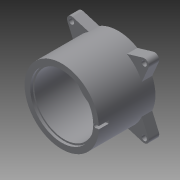
# Autodesk Inventor part: Nikon Mount 02
Saved by Autodesk Inventor 2013 (Build 170138000, 138)
## iProperties
Created: 2014-04-13
Part Number: Nikon Mount 02
Material: Generic
Document SubType Name: Modeling
Designer: spichelh
Density: 1 g/cm^3
Author: spichelh
Autodesk Inventor part; units mm, degrees
ref_plane "YZ Plane" through (0, 0, 0) normal (1, 0, 0) x (0, 1, 0)
ref_plane "XZ Plane" through (0, 0, 0) normal (0, 1, 0) x (-1, 0, 0)
ref_plane "XY Plane" through (0, 0, 0) normal (0, 0, 1) x (1, 0, 0)
sketch "Sketch1" plane through (0, 0, 0) normal (0, 0, 1) x (1, 0, 0)
  circle A0 centre (0.0056, 55.7001) radius 1.4
  arc A1 (1.0027, 59.055) -> (-3.2054, 54.3074) centre (0.0056, 55.7001) ccw
  circle A2 centre (27.9456, 30.9351) radius 20
  line L0 (27.9456, 30.9351) -> (77.9456, 30.9351) construction
  line L1 (27.9456, 30.9351) -> (77.9456, 30.9351) construction
  line L2 (1.0027, 59.055) -> (13.3178, 55.3948)
  line L3 (-3.2054, 54.3074) -> (1.9067, 42.5207)
  circle A3 centre (0.0056, 6.1701) radius 1.4
  circle A4 centre (55.8856, 6.1701) radius 1.4
  line L4 (55.8856, 55.7001) -> (0.0056, 6.1701) construction
  line L5 (55.8856, 6.1701) -> (0.0056, 55.7001) construction
  line L6 (27.9456, 30.9351) -> (27.9456, 40.8752) construction
  line L7 (27.9456, 30.9351) -> (19.6856, 30.9351) construction
  arc A5 (59.0966, 54.3074) -> (54.8884, 59.055) centre (55.8856, 55.7001) ccw
  line L8 (54.8884, 59.055) -> (42.5733, 55.3948)
  line L9 (59.0966, 54.3074) -> (53.9844, 42.5207)
  circle A6 centre (55.8856, 55.7001) radius 1.4
  arc A7 (42.5733, 55.3948) -> (13.3178, 55.3948) centre (27.9456, 30.9351) ccw
  arc A8 (1.9067, 42.5207) -> (53.9844, 42.5207) centre (27.9456, 30.9351) ccw construction
  arc A9 (42.5733, 55.3948) -> (13.3178, 55.3948) centre (27.9456, 30.9351) ccw construction
  arc A10 (-3.2054, 7.5627) -> (1.0027, 2.8151) centre (0.0056, 6.1701) ccw
  line L10 (1.0027, 2.8151) -> (13.3178, 6.4753)
  line L11 (-3.2054, 7.5627) -> (1.9067, 19.3494)
  arc A11 (54.8884, 2.8151) -> (59.0966, 7.5627) centre (55.8856, 6.1701) ccw
  line L12 (54.8884, 2.8151) -> (42.5733, 6.4753)
  line L13 (59.0966, 7.5627) -> (53.9844, 19.3494)
  arc A12 (53.9844, 19.3494) -> (53.9844, 42.5207) centre (27.9456, 30.9351) ccw
  arc A13 (1.9067, 42.5207) -> (1.9067, 19.3494) centre (27.9456, 30.9351) ccw
  arc A14 (13.3178, 6.4753) -> (42.5733, 6.4753) centre (27.9456, 30.9351) ccw
  point P0 (0, 0)
  point P1 (27.9456, 30.9351)
  dimension "d222" = 2.8
  dimension "d223" = 7
  dimension "d233" = 40
  dimension "d234" = 27.9456
  dimension "d291" = 55.88
  dimension "d292" = 49.53
  dimension "d293" = 2.8
  dimension "d294" = 2.8
  dimension "d295" = 155
  dimension "d296" = 155
  dimension "d298" = 30.9351
  dimension "d299" = 28.5
  dimension "d300" = 155
  dimension "d301" = 3.5
  dimension "d302" = 155
  dimension "d303" = 28.5
  constraints: 28 end point, 22 point on circle, 15 centre point, 10 symmetric about line, 6 coincident, 4 tangent, 2 horizontal, 2 horizontal alignment, 2 midpoint, 2 perpendicular, 2 vertical alignment, 3 other
  measures "d222" diameter of A0
  measures "d223" diameter of A1
  measures "d233" diameter of A2
  measures "d234" horizontal distance of L0.start point (0, 0)
  measures "d291" distance of A0.centre L4.start
  measures "d292" distance of point (0.006, 6.17) A0.centre
  measures "d293" diameter of A3
  measures "d294" diameter of A4
  measures "d295" angle of L5 L2
  measures "d296" angle of L5 L3
  measures "d298" vertical distance of point (0, 0) A8.centre
  measures "d299" radius of A7
  measures "d300" angle of L10 L4
  measures "d301" radius of A10
  measures "d302" angle of L4 L11
  measures "d303" radius of A12
extrude "Extrusion1" add sketch "Sketch1" along normal blind 8
sketch "Sketch14" plane through (0, 0, 8) normal (0, 0, 1) x (1, 0, 0)
  circle A0 centre (27.9456, 30.9351) radius 23
  line L0 (27.9493, 53.53) -> (27.94, -2.5) construction
  line L1 (50.88, 56.34) -> (5, 56.34) construction
  line L2 (-22.86, -0.81) -> (78.74, -0.81) construction
  line L3 (-22.86, 56.34) -> (-22.86, -0.81) construction
  line L4 (78.74, -0.81) -> (78.74, 56.34) construction
  circle A1 centre (27.9456, 30.9351) radius 20 projected
  arc A2 (42.5733, 55.3948) -> (13.3178, 55.3948) centre (27.9456, 30.9351) ccw projected
  circle A3 centre (27.9456, 30.9351) radius 28.5
  point P0 (52.88, -2.5)
  dimension "d96" = 46
  constraints: 2 centre point, 2 coincident, 2 end point, 1 concentric, 1 point on line
  measures "d96" diameter of A0
extrude "Extrusion14" add sketch "Sketch14" against normal blind 8 contours A3 A2
sketch "Sketch15" plane through (0, 0, 8) normal (0, 0, 1) x (1, 0, 0)
  circle A0 centre (27.9456, 30.9351) radius 20 projected
  circle A1 centre (27.9456, 30.9351) radius 28.5
  circle A2 centre (27.9456, 30.9351) radius 23
  dimension "d306" = 46
  dimension "d307" = 57
  constraints: 3 coincident, 2 centre point
  measures "d306" diameter of A2
  measures "d307" diameter of A1
extrude "Extrusion15" add sketch "Sketch15" along normal blind 35.44 contours A1
sketch "Sketch41" plane through (0, 0, 8) normal (0, 0, 1) x (1, 0, 0)
  arc A0 (55.6663, 24.3163) -> (0.2017, 24.4136) centre (27.94, 27.765) ccw projected
  circle A1 centre (0.0056, 55.7001) radius 1.4 projected
  circle A2 centre (0.0056, 55.7001) radius 2
  line L0 (27.94, 27.765) -> (27.94, 38.7432) construction
  line L1 (27.94, 27.765) -> (35.7476, 27.765) construction
  circle A3 centre (55.8744, 55.7001) radius 2
  circle A4 centre (0.0056, 6.1701) radius 1.4 projected
  circle A5 centre (55.8856, 6.1701) radius 1.4 projected
  circle A6 centre (0.0056, 6.1701) radius 2
  circle A7 centre (55.8856, 6.1701) radius 2
  point P0 (3.5123, 41.3272)
  point P1 (14.3575, 52.1814)
  point P2 (0, 0)
  dimension "d287" = 4
  dimension "d304" = 4
  dimension "d305" = 4
  constraints: 4 centre point, 4 end point, 3 coincident, 1 perpendicular, 1 symmetric about line, 1 vertical, 1 other
  measures "d287" diameter of A2
  measures "d304" diameter of A6
  measures "d305" diameter of A7
extrude "Extrusion39" cut sketch "Sketch41" against normal blind 4 contours A1 | A2 | A3 | A4 | A6 | A7
sketch "Sketch17" plane through (0, 0, 0) normal (0, 0, -1) x (-1, 0, 0)
  line L0 (-37.3456, 38.9851) -> (-18.5456, 38.9851)
  line L1 (-17.5456, 37.9851) -> (-17.5456, 23.8851)
  line L2 (-18.5456, 22.8851) -> (-37.3456, 22.8851)
  line L3 (-38.3456, 23.8851) -> (-38.3456, 37.9851)
  line L4 (-17.5456, 38.9851) -> (-38.3456, 22.8851) construction
  line L5 (-17.5456, 22.8851) -> (-38.3456, 38.9851) construction
  circle A0 centre (-27.9456, 30.9351) radius 23
  arc A1 (-37.3456, 38.9851) -> (-38.3456, 37.9851) centre (-37.3456, 37.9851) ccw
  arc A2 (-38.3456, 23.8851) -> (-37.3456, 22.8851) centre (-37.3456, 23.8851) ccw
  arc A3 (-18.5456, 22.8851) -> (-17.5456, 23.8851) centre (-18.5456, 23.8851) ccw
  arc A4 (-17.5456, 37.9851) -> (-18.5456, 38.9851) centre (-18.5456, 37.9851) ccw
  circle A5 centre (-27.9456, 30.9351) radius 20 projected
  point P0 (0, 0)
  point P1 (-27.9456, 30.9351)
  dimension "d111" = 20.8
  dimension "d112" = 16.1
  dimension "d115" = 1
  dimension "d308" = 46
  constraints: 12 end point, 8 point on circle, 8 point on line, 8 tangent, 5 centre point, 3 equal radius, 2 coincident, 2 midpoint, 2 parallel, 1 horizontal, 1 perpendicular
  measures "d111" distance of L5.start L4.end
  measures "d112" distance of L4.start L5.start
  measures "d115" radius of A1
  measures "d308" diameter of A0
extrude "Extrusion17" add sketch "Sketch17" against normal blind 11 contours A0 | A5
sketch "Sketch18" plane through (27.94, 27.765, 11) normal (0, 0, 1) x (1, 0, 0)
  line L0 (10.4056, 10.2201) -> (10.4056, -3.8799) projected
  line L1 (9.4056, -4.8799) -> (-9.3944, -4.8799) projected
  line L2 (-10.3944, -3.8799) -> (-10.3944, 10.2201) projected
  line L3 (-9.3944, 11.2201) -> (9.4056, 11.2201) projected
  arc A0 (10.4056, 10.2201) -> (9.4056, 11.2201) centre (9.4056, 10.2201) ccw projected
  arc A1 (9.4056, -4.8799) -> (10.4056, -3.8799) centre (9.4056, -3.8799) ccw projected
  arc A2 (-10.3944, -3.8799) -> (-9.3944, -4.8799) centre (-9.3944, -3.8799) ccw projected
  arc A3 (-9.3944, 11.2201) -> (-10.3944, 10.2201) centre (-9.3944, 10.2201) ccw projected
  line L4 (9.4056, 12.2201) -> (-9.3944, 12.2201)
  arc A4 (-9.3944, 12.2201) -> (-11.3944, 10.2201) centre (-9.3944, 10.2201) ccw
  line L5 (-11.3944, 10.2201) -> (-11.3944, -3.8799)
  arc A5 (-11.3944, -3.8799) -> (-9.3944, -5.8799) centre (-9.3944, -3.8799) ccw
  line L6 (-9.3944, -5.8799) -> (9.4056, -5.8799)
  arc A6 (9.4056, -5.8799) -> (11.4056, -3.8799) centre (9.4056, -3.8799) ccw
  line L7 (11.4056, -3.8799) -> (11.4056, 10.2201)
  arc A7 (11.4056, 10.2201) -> (9.4056, 12.2201) centre (9.4056, 10.2201) ccw
  point P0 (10.4, 8.05)
  point P1 (10.4, -8.05)
  point P2 (-10.4, -8.05)
  point P3 (-10.4, 8.05)
  point P4 (-27.94, -27.765)
  dimension "d116" = 1
  constraints: 8 end point, 8 point on circle, 4 centre point, 11 other
extrude "Extrusion18" cut sketch "Sketch18" against normal blind 8
sketch "Sketch19" plane through (27.94, 27.765, 11) normal (0, 0, 1) x (1, 0, 0)
  arc A0 (-9.3944, 12.2201) -> (-11.3944, 10.2201) centre (-9.3944, 10.2201) ccw projected
  line L0 (-9.3944, 12.2201) -> (9.4056, 12.2201) projected
  arc A1 (11.4056, 10.2201) -> (9.4056, 12.2201) centre (9.4056, 10.2201) ccw projected
  line L1 (11.4056, 10.2201) -> (11.4056, -3.8799) projected
  arc A2 (9.4056, -5.8799) -> (11.4056, -3.8799) centre (9.4056, -3.8799) ccw projected
  line L2 (9.4056, -5.8799) -> (-9.3944, -5.8799) projected
  arc A3 (-11.3944, -3.8799) -> (-9.3944, -5.8799) centre (-9.3944, -3.8799) ccw projected
  line L3 (-11.3944, -3.8799) -> (-11.3944, 10.2201) projected
  line L4 (9.4056, 13.2201) -> (-9.3944, 13.2201)
  arc A4 (-9.3944, 13.2201) -> (-12.3944, 10.2201) centre (-9.3944, 10.2201) ccw
  line L5 (-12.3944, 10.2201) -> (-12.3944, -3.8799)
  arc A5 (-12.3944, -3.8799) -> (-9.3944, -6.8799) centre (-9.3944, -3.8799) ccw
  line L6 (-9.3944, -6.8799) -> (9.4056, -6.8799)
  arc A6 (9.4056, -6.8799) -> (12.4056, -3.8799) centre (9.4056, -3.8799) ccw
  line L7 (12.4056, -3.8799) -> (12.4056, 10.2201)
  arc A7 (12.4056, 10.2201) -> (9.4056, 13.2201) centre (9.4056, 10.2201) ccw
  point P0 (-27.94, -27.765)
  dimension "d119" = 1
  constraints: 8 end point, 8 point on circle, 4 centre point, 7 other
  measures "d119" distance between parallel lines of L0 L4
extrude "Extrusion19" cut sketch "Sketch19" against normal blind 7
sketch "Sketch20" plane through (27.94, 27.765, 11) normal (0, 0, 1) x (1, 0, 0)
  arc A0 (-9.3944, 13.2201) -> (-12.3944, 10.2201) centre (-9.3944, 10.2201) ccw projected
  line L0 (-9.3944, 13.2201) -> (9.4056, 13.2201) projected
  arc A1 (12.4056, 10.2201) -> (9.4056, 13.2201) centre (9.4056, 10.2201) ccw projected
  line L1 (12.4056, 10.2201) -> (12.4056, -3.8799) projected
  arc A2 (9.4056, -6.8799) -> (12.4056, -3.8799) centre (9.4056, -3.8799) ccw projected
  line L2 (9.4056, -6.8799) -> (-9.3944, -6.8799) projected
  arc A3 (-12.3944, -3.8799) -> (-9.3944, -6.8799) centre (-9.3944, -3.8799) ccw projected
  line L3 (-12.3944, -3.8799) -> (-12.3944, 10.2201) projected
  line L4 (9.4056, 14.2201) -> (-9.3944, 14.2201)
  arc A4 (-9.3944, 14.2201) -> (-13.3944, 10.2201) centre (-9.3944, 10.2201) ccw
  line L5 (-13.3944, 10.2201) -> (-13.3944, -3.8799)
  arc A5 (-13.3944, -3.8799) -> (-9.3944, -7.8799) centre (-9.3944, -3.8799) ccw
  line L6 (-9.3944, -7.8799) -> (9.4056, -7.8799)
  arc A6 (9.4056, -7.8799) -> (13.4056, -3.8799) centre (9.4056, -3.8799) ccw
  line L7 (13.4056, -3.8799) -> (13.4056, 10.2201)
  arc A7 (13.4056, 10.2201) -> (9.4056, 14.2201) centre (9.4056, 10.2201) ccw
  point P0 (-27.94, -27.765)
  dimension "d122" = 1
  constraints: 8 end point, 8 point on circle, 4 centre point, 7 other
  measures "d122" distance between parallel lines of L4 L0
extrude "Extrusion20" cut sketch "Sketch20" against normal blind 6
sketch "Sketch21" plane through (27.94, 27.765, 11) normal (0, 0, 1) x (1, 0, 0)
  arc A0 (-9.3944, 14.2201) -> (-13.3944, 10.2201) centre (-9.3944, 10.2201) ccw projected
  line L0 (-9.3944, 14.2201) -> (9.4056, 14.2201) projected
  arc A1 (13.4056, 10.2201) -> (9.4056, 14.2201) centre (9.4056, 10.2201) ccw projected
  line L1 (13.4056, 10.2201) -> (13.4056, -3.8799) projected
  arc A2 (9.4056, -7.8799) -> (13.4056, -3.8799) centre (9.4056, -3.8799) ccw projected
  line L2 (9.4056, -7.8799) -> (-9.3944, -7.8799) projected
  arc A3 (-13.3944, -3.8799) -> (-9.3944, -7.8799) centre (-9.3944, -3.8799) ccw projected
  line L3 (-13.3944, -3.8799) -> (-13.3944, 10.2201) projected
  line L4 (9.4056, 15.2201) -> (-9.3944, 15.2201)
  arc A4 (-9.3944, 15.2201) -> (-14.3944, 10.2201) centre (-9.3944, 10.2201) ccw
  line L5 (-14.3944, 10.2201) -> (-14.3944, -3.8799)
  arc A5 (-14.3944, -3.8799) -> (-9.3944, -8.8799) centre (-9.3944, -3.8799) ccw
  line L6 (-9.3944, -8.8799) -> (9.4056, -8.8799)
  arc A6 (9.4056, -8.8799) -> (14.4056, -3.8799) centre (9.4056, -3.8799) ccw
  line L7 (14.4056, -3.8799) -> (14.4056, 10.2201)
  arc A7 (14.4056, 10.2201) -> (9.4056, 15.2201) centre (9.4056, 10.2201) ccw
  point P0 (-27.94, -27.765)
  dimension "d125" = 1
  constraints: 8 end point, 8 point on circle, 4 centre point, 7 other
  measures "d125" distance between parallel lines of L0 L4
extrude "Extrusion21" cut sketch "Sketch21" against normal blind 5
sketch "Sketch22" plane through (27.94, 27.765, 11) normal (0, 0, 1) x (1, 0, 0)
  arc A0 (-9.3944, 15.2201) -> (-14.3944, 10.2201) centre (-9.3944, 10.2201) ccw projected
  line L0 (-9.3944, 15.2201) -> (9.4056, 15.2201) projected
  arc A1 (14.4056, 10.2201) -> (9.4056, 15.2201) centre (9.4056, 10.2201) ccw projected
  line L1 (14.4056, 10.2201) -> (14.4056, -3.8799) projected
  arc A2 (9.4056, -8.8799) -> (14.4056, -3.8799) centre (9.4056, -3.8799) ccw projected
  line L2 (9.4056, -8.8799) -> (-9.3944, -8.8799) projected
  arc A3 (-14.3944, -3.8799) -> (-9.3944, -8.8799) centre (-9.3944, -3.8799) ccw projected
  line L3 (-14.3944, -3.8799) -> (-14.3944, 10.2201) projected
  line L4 (9.4056, 16.2201) -> (-9.3944, 16.2201)
  arc A4 (-9.3944, 16.2201) -> (-15.3944, 10.2201) centre (-9.3944, 10.2201) ccw
  line L5 (-15.3944, 10.2201) -> (-15.3944, -3.8799)
  arc A5 (-15.3944, -3.8799) -> (-9.3944, -9.8799) centre (-9.3944, -3.8799) ccw
  line L6 (-9.3944, -9.8799) -> (9.4056, -9.8799)
  arc A6 (9.4056, -9.8799) -> (15.4056, -3.8799) centre (9.4056, -3.8799) ccw
  line L7 (15.4056, -3.8799) -> (15.4056, 10.2201)
  arc A7 (15.4056, 10.2201) -> (9.4056, 16.2201) centre (9.4056, 10.2201) ccw
  point P0 (-27.94, -27.765)
  dimension "d128" = 1
  constraints: 8 end point, 8 point on circle, 4 centre point, 7 other
  measures "d128" distance between parallel lines of L0 L4
extrude "Extrusion22" cut sketch "Sketch22" against normal blind 4
sketch "Sketch23" plane through (27.94, 27.765, 11) normal (0, 0, 1) x (1, 0, 0)
  arc A0 (-9.3944, 16.2201) -> (-15.3944, 10.2201) centre (-9.3944, 10.2201) ccw projected
  line L0 (-9.3944, 16.2201) -> (9.4056, 16.2201) projected
  arc A1 (15.4056, 10.2201) -> (9.4056, 16.2201) centre (9.4056, 10.2201) ccw projected
  line L1 (15.4056, 10.2201) -> (15.4056, -3.8799) projected
  arc A2 (9.4056, -9.8799) -> (15.4056, -3.8799) centre (9.4056, -3.8799) ccw projected
  line L2 (9.4056, -9.8799) -> (-9.3944, -9.8799) projected
  arc A3 (-15.3944, -3.8799) -> (-9.3944, -9.8799) centre (-9.3944, -3.8799) ccw projected
  line L3 (-15.3944, -3.8799) -> (-15.3944, 10.2201) projected
  line L4 (9.4056, 17.2201) -> (-9.3944, 17.2201)
  arc A4 (-9.3944, 17.2201) -> (-16.3944, 10.2201) centre (-9.3944, 10.2201) ccw
  line L5 (-16.3944, 10.2201) -> (-16.3944, -3.8799)
  arc A5 (-16.3944, -3.8799) -> (-9.3944, -10.8799) centre (-9.3944, -3.8799) ccw
  line L6 (-9.3944, -10.8799) -> (9.4056, -10.8799)
  arc A6 (9.4056, -10.8799) -> (16.4056, -3.8799) centre (9.4056, -3.8799) ccw
  line L7 (16.4056, -3.8799) -> (16.4056, 10.2201)
  arc A7 (16.4056, 10.2201) -> (9.4056, 17.2201) centre (9.4056, 10.2201) ccw
  point P0 (-27.94, -27.765)
  dimension "d131" = 1
  constraints: 8 end point, 8 point on circle, 4 centre point, 7 other
  measures "d131" distance between parallel lines of L0 L4
extrude "Extrusion23" cut sketch "Sketch23" against normal blind 3
sketch "Sketch24" plane through (27.94, 27.765, 11) normal (0, 0, 1) x (1, 0, 0)
  arc A0 (-9.3944, 17.2201) -> (-16.3944, 10.2201) centre (-9.3944, 10.2201) ccw projected
  line L0 (-9.3944, 17.2201) -> (9.4056, 17.2201) projected
  arc A1 (16.4056, 10.2201) -> (9.4056, 17.2201) centre (9.4056, 10.2201) ccw projected
  line L1 (16.4056, 10.2201) -> (16.4056, -3.8799) projected
  arc A2 (9.4056, -10.8799) -> (16.4056, -3.8799) centre (9.4056, -3.8799) ccw projected
  line L2 (9.4056, -10.8799) -> (-9.3944, -10.8799) projected
  arc A3 (-16.3944, -3.8799) -> (-9.3944, -10.8799) centre (-9.3944, -3.8799) ccw projected
  line L3 (-16.3944, -3.8799) -> (-16.3944, 10.2201) projected
  line L4 (9.4056, 18.2201) -> (-9.3944, 18.2201)
  arc A4 (-9.3944, 18.2201) -> (-17.3944, 10.2201) centre (-9.3944, 10.2201) ccw
  line L5 (-17.3944, 10.2201) -> (-17.3944, -3.8799)
  arc A5 (-17.3944, -3.8799) -> (-9.3944, -11.8799) centre (-9.3944, -3.8799) ccw
  line L6 (-9.3944, -11.8799) -> (9.4056, -11.8799)
  arc A6 (9.4056, -11.8799) -> (17.4056, -3.8799) centre (9.4056, -3.8799) ccw
  line L7 (17.4056, -3.8799) -> (17.4056, 10.2201)
  arc A7 (17.4056, 10.2201) -> (9.4056, 18.2201) centre (9.4056, 10.2201) ccw
  point P0 (-27.94, -27.765)
  dimension "d134" = 1
  constraints: 8 end point, 8 point on circle, 4 centre point, 7 other
  measures "d134" distance between parallel lines of L0 L4
extrude "Extrusion24" cut sketch "Sketch24" against normal blind 2
sketch "Sketch25" plane through (27.94, 27.765, 11) normal (0, 0, 1) x (1, 0, 0)
  arc A0 (-9.3944, 18.2201) -> (-17.3944, 10.2201) centre (-9.3944, 10.2201) ccw projected
  line L0 (-9.3944, 18.2201) -> (9.4056, 18.2201) projected
  arc A1 (17.4056, 10.2201) -> (9.4056, 18.2201) centre (9.4056, 10.2201) ccw projected
  line L1 (17.4056, 10.2201) -> (17.4056, -3.8799) projected
  arc A2 (9.4056, -11.8799) -> (17.4056, -3.8799) centre (9.4056, -3.8799) ccw projected
  line L2 (9.4056, -11.8799) -> (-9.3944, -11.8799) projected
  arc A3 (-17.3944, -3.8799) -> (-9.3944, -11.8799) centre (-9.3944, -3.8799) ccw projected
  line L3 (-17.3944, -3.8799) -> (-17.3944, 10.2201) projected
  line L4 (9.4056, 19.2201) -> (-9.3944, 19.2201)
  arc A4 (-9.3944, 19.2201) -> (-18.3944, 10.2201) centre (-9.3944, 10.2201) ccw
  line L5 (-18.3944, 10.2201) -> (-18.3944, -3.8799)
  arc A5 (-18.3944, -3.8799) -> (-9.3944, -12.8799) centre (-9.3944, -3.8799) ccw
  line L6 (-9.3944, -12.8799) -> (9.4056, -12.8799)
  arc A6 (9.4056, -12.8799) -> (18.4056, -3.8799) centre (9.4056, -3.8799) ccw
  line L7 (18.4056, -3.8799) -> (18.4056, 10.2201)
  arc A7 (18.4056, 10.2201) -> (9.4056, 19.2201) centre (9.4056, 10.2201) ccw
  point P0 (-27.94, -27.765)
  dimension "d137" = 1
  constraints: 8 end point, 8 point on circle, 4 centre point, 7 other
  measures "d137" distance between parallel lines of L0 L4
extrude "Extrusion25" cut sketch "Sketch25" against normal blind 1
sketch "Sketch39" plane through (0, 0, 0) normal (0, 0, -1) x (-1, 0, 0)
  arc A0 (-38.3456, 23.8851) -> (-37.3456, 22.8851) centre (-37.3456, 23.8851) ccw projected
  line L0 (-38.3456, 23.8851) -> (-38.3456, 37.9851) projected
  arc A1 (-37.3456, 38.9851) -> (-38.3456, 37.9851) centre (-37.3456, 37.9851) ccw projected
  line L1 (-37.3456, 38.9851) -> (-18.5456, 38.9851) projected
  arc A2 (-17.5456, 37.9851) -> (-18.5456, 38.9851) centre (-18.5456, 37.9851) ccw projected
  line L2 (-17.5456, 37.9851) -> (-17.5456, 23.8851) projected
  arc A3 (-18.5456, 22.8851) -> (-17.5456, 23.8851) centre (-18.5456, 23.8851) ccw projected
  line L3 (-18.5456, 22.8851) -> (-37.3456, 22.8851) projected
  line L4 (-40.4456, 43.4351) -> (-15.4456, 43.4351)
  line L5 (-15.4456, 43.4351) -> (-15.4456, 18.4351)
  line L6 (-15.4456, 18.4351) -> (-40.4456, 18.4351)
  line L7 (-40.4456, 18.4351) -> (-40.4456, 43.4351)
  line L8 (-15.4456, 43.4351) -> (-40.4456, 18.4351) construction
  line L9 (-40.4456, 43.4351) -> (-15.4456, 18.4351) construction
  line L10 (-18.5456, 23.8851) -> (-37.3456, 37.9851) construction
  line L11 (-37.3456, 23.8851) -> (-18.5456, 37.9851) construction
  point P0 (-27.9456, 30.9351)
  dimension "d217" = 25
  dimension "d219" = 25
  constraints: 16 end point, 3 midpoint, 2 parallel, 1 horizontal, 1 perpendicular
  measures "d217" distance of L4.start L4.end
  measures "d219" distance of L4.end L5.end
extrude "Extrusion38" cut sketch "Sketch39" against normal blind 1.6
sketch "Sketch40" plane through (0, 0, 1.6) normal (0, 0, -1) x (-1, 0, 0)
  line L0 (-37.3456, 22.8851) -> (-18.5456, 22.8851) projected
  arc A0 (-38.3456, 23.8851) -> (-37.3456, 22.8851) centre (-37.3456, 23.8851) ccw projected
  line L1 (-38.3456, 37.9851) -> (-38.3456, 23.8851) projected
  arc A1 (-37.3456, 38.9851) -> (-38.3456, 37.9851) centre (-37.3456, 37.9851) ccw projected
  line L2 (-18.5456, 38.9851) -> (-37.3456, 38.9851) projected
  arc A2 (-17.5456, 37.9851) -> (-18.5456, 38.9851) centre (-18.5456, 37.9851) ccw projected
  line L3 (-17.5456, 23.8851) -> (-17.5456, 37.9851) projected
  arc A3 (-18.5456, 22.8851) -> (-17.5456, 23.8851) centre (-18.5456, 23.8851) ccw projected
  line L4 (-40.4456, 43.4351) -> (-15.4456, 43.4351) projected
  line L5 (-40.4456, 18.4351) -> (-40.4456, 43.4351) projected
  line L6 (-15.4456, 18.4351) -> (-40.4456, 18.4351) projected
  line L7 (-15.4456, 43.4351) -> (-15.4456, 18.4351) projected
  line L8 (-15.4456, 43.4351) -> (-40.4456, 18.4351) construction
  line L9 (-15.4456, 18.4351) -> (-40.4456, 43.4351) construction
  point P0 (0, 0)
  point P1 (-27.9456, 30.9351)
  constraints: 4 end point, 1 midpoint, 1 perpendicular
sketch "Sketch42" plane through (27.9456, 30.9351, 43.44) normal (0, 0, 1) x (1, 0, 0)
  circle A0 centre (0, 0) radius 23 projected
  circle A1 centre (0, 0) radius 28.5 projected
  circle A2 centre (0, 0) radius 24.2
  point P0 (-27.9456, -30.9351)
  dimension "d310" = 48.4
  constraints: 1 centre point, 1 coincident
  measures "d310" diameter of A2
extrude "Extrusion40" cut sketch "Sketch42" against normal blind 2 contours A2
sketch "Sketch43" plane through (27.9456, 30.9351, 43.44) normal (0, 0, 1) x (1, 0, 0)
  circle A0 centre (26, 0) radius 1.5
  circle A1 centre (0, 0) radius 24.2 projected
  circle A2 centre (0, 0) radius 28.5 projected
  line L0 (27.0198, -1.1) -> (29, -1.1)
  line L1 (29, -1.1) -> (29, 1.1)
  line L2 (29, 1.1) -> (27.0198, 1.1)
  line L3 (0, 0) -> (33.1676, 0) construction
  line L4 (29, 0) -> (29.3811, 0) construction
  point P0 (-27.9456, -30.9351)
  dimension "d315" = 3
  dimension "d317" = 26
  dimension "d318" = 3
  dimension "d319" = 2.2
  dimension "d320" = 4
  constraints: 10 end point, 2 collinear, 2 parallel, 2 point on circle, 1 centre point, 1 horizontal, 1 midpoint, 1 perpendicular, 1 point on line
  measures "d315" diameter of A0
  measures "d317" distance of A1.centre A0.centre
  measures "d318" distance from line of L1 A0.centre
  measures "d319" distance of L0.end L1.end
extrude "Extrusion41" cut sketch "Sketch43" against normal blind 7.6 contours A0 | A0 L2 A2 L0 | L2 L1 L0 A2 picked at (28.1147, -0.8112)
sketch "Sketch44" plane through (27.9456, 30.9351, 35.84) normal (0, 0, 1) x (1, 0, 0)
  arc A0 (27.0198, 1.1) -> (27.0198, -1.1) centre (26, 0) ccw projected
  circle A1 centre (26, 0) radius 0.65
  point P0 (-27.9456, -30.9351)
  dimension "d321" = 1.3
  constraints: 1 centre point, 1 coincident
  measures "d321" diameter of A1
extrude "Extrusion42" cut sketch "Sketch44" against normal blind 3
body "Solid1"
